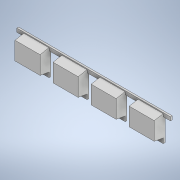
# Autodesk Inventor part: Buttons
Saved by Autodesk Inventor 2020 (Build 240168000, 168)
## iProperties
Created: 2022-03-19
Part Number: Buttons
Material: Типовые
Document SubType Name: Modeling
Designer: NoName
Density: 1 g/cm^3
Appearance: По умолчанию
Author: NoName
Autodesk Inventor part; units mm, degrees
ref_plane "YZ Plane" through (0, 0, 0) normal (1, 0, 0) x (0, 1, 0)
ref_plane "XZ Plane" through (0, 0, 0) normal (0, 1, 0) x (-1, 0, 0)
ref_plane "XY Plane" through (0, 0, 0) normal (0, 0, 1) x (1, 0, 0)
sketch "Эскиз1" plane through (0, 0, 0) normal (0, 0, 1) x (1, 0, 0)
  line L0 (0, 0) -> (5.6, 0)
  line L1 (5.6, 0) -> (5.6, 6)
  line L2 (5.6, 6) -> (0, 6)
  line L3 (0, 6) -> (0, 0)
  line L4 (8.5, 0) -> (14.1, 0)
  line L5 (14.1, 0) -> (14.1, 6)
  line L6 (14.1, 6) -> (8.5, 6)
  line L7 (8.5, 6) -> (8.5, 0)
  line L8 (17, 0) -> (22.6, 0)
  line L9 (22.6, 0) -> (22.6, 6)
  line L10 (22.6, 6) -> (17, 6)
  line L11 (17, 6) -> (17, 0)
  line L12 (25.5, 0) -> (31.1, 0)
  line L13 (31.1, 0) -> (31.1, 6)
  line L14 (31.1, 6) -> (25.5, 6)
  line L15 (25.5, 6) -> (25.5, 0)
  line L16 (5.6, 6) -> (8.5, 6)
  line L17 (14.1, 6) -> (17, 6)
  line L18 (22.6, 6) -> (25.5, 6)
  line L19 (22.6, 5.2) -> (25.5, 5.2)
  line L20 (17, 5.2) -> (14.1, 5.2)
  line L21 (8.5, 5.2) -> (5.6, 5.2)
  line L22 (0, 5.2) -> (-1.6, 5.2)
  line L23 (-1.6, 5.2) -> (-1.6, 6)
  line L24 (-1.6, 6) -> (0, 6)
  line L25 (0, 6) -> (0, 5.2)
  line L26 (31.1, 5.2) -> (32.7, 5.2)
  line L27 (32.7, 5.2) -> (32.7, 6)
  line L28 (32.7, 6) -> (31.1, 6)
  line L29 (31.1, 6) -> (31.1, 5.2)
  dimension "d0" = 5.6
  dimension "d1" = 6
  dimension "d4" = 8.5
  dimension "d9" = 0.8
  dimension "d10" = 1.6
  constraints: 60 end point, 11 point on line, 6 parallel, 5 horizontal, 5 perpendicular, 4 collinear, 4 horizontal alignment, 23 other
  measures "d0" distance between parallel lines of L3 L1
  measures "d1" distance between parallel lines of L0 L2
  measures "d4" distance of L0.start L4.start
  measures "d9" distance between parallel lines of L16 L21
  measures "d10" distance between parallel lines of L3 L23
extrude "Выдавливание1" add sketch "Эскиз1" along normal blind 0.4
sketch "Эскиз2" plane through (0, 0, 0.4) normal (0, 0, 1) x (1, 0, 0)
  line L0 (0, 5.2) -> (0, 0) projected
  line L1 (5.6, 0) -> (5.6, 5.2) projected
  line L2 (0, 1.1) -> (5.6, 1.1)
  line L3 (5.6, 1.1) -> (5.6, 5.8)
  line L4 (5.6, 5.8) -> (0, 5.8)
  line L5 (0, 5.8) -> (0, 1.1)
  line L6 (8.5, 5.2) -> (8.5, 0) projected
  line L7 (14.1, 0) -> (14.1, 5.2) projected
  line L8 (8.5, 1.1) -> (14.1, 1.1)
  line L9 (14.1, 1.1) -> (14.1, 5.8)
  line L10 (14.1, 5.8) -> (8.5, 5.8)
  line L11 (8.5, 5.8) -> (8.5, 1.1)
  line L12 (17, 5.2) -> (17, 0) projected
  line L13 (22.6, 0) -> (22.6, 5.2) projected
  line L14 (17, 1.1) -> (22.6, 1.1)
  line L15 (22.6, 1.1) -> (22.6, 5.8)
  line L16 (22.6, 5.8) -> (17, 5.8)
  line L17 (17, 5.8) -> (17, 1.1)
  line L18 (25.5, 5.2) -> (25.5, 0) projected
  line L19 (31.1, 0) -> (31.1, 5.2) projected
  line L20 (25.5, 1.1) -> (31.1, 1.1)
  line L21 (31.1, 1.1) -> (31.1, 5.8)
  line L22 (31.1, 5.8) -> (25.5, 5.8)
  line L23 (25.5, 5.8) -> (25.5, 1.1)
  line L24 (0, 0) -> (5.6, 0) projected
  point P0 (25.5, 5)
  point P1 (17, 5)
  point P2 (8.5, 5)
  point P3 (0, 5)
  dimension "d13" = 1.1
  dimension "d14" = 4.7
  constraints: 32 end point, 14 point on line, 8 parallel, 4 horizontal, 4 perpendicular
  measures "d13" distance between parallel lines of L24 L2
  measures "d14" distance between parallel lines of L2 L4
extrude "Выдавливание2" add sketch "Эскиз2" along normal blind 2 contours L5 L4 L3 L1 L2 L0 | L11 L10 L9 L7 L8 L6 | L17 L16 L15 L13 L14 L12 | L23 L22 L21 L19 L20 L18
sketch "Эскиз3" plane through (0, 0, 0) normal (-1, 0, 0) x (0, 0, 1)
  line L0 (0.4, 1.1) -> (2.4, 1.45)
  line L1 (0, 5.2) -> (0, 0) projected
  line L2 (0, 0) -> (0.4, 0) projected
  line L3 (0.4, 1.1) -> (0.4, 0) projected
  line L4 (0.4, 1.1) -> (2.4, 1.1) projected
  line L5 (2.4, 5.8) -> (2.4, 1.1) projected
  line L6 (0.4, 5.2) -> (0.4, 5.8) projected
  line L7 (0, 5.2) -> (0.4, 5.2) projected
  line L8 (0.4, 1.1) -> (2.4, 1.1)
  line L9 (0.4, 5.8) -> (2.4, 5.8)
  line L10 (0.4, 5.8) -> (2.4, 5.45)
  line L11 (2.4, 1.1) -> (2.4, 5.8) projected
  line L12 (2.4, 1.45) -> (2.4, 1.1)
  line L13 (0.4, 5.8) -> (2.4, 5.8) projected
  line L14 (0.4, 6) -> (0.4, 5.2) projected
  line L15 (2.4, 5.8) -> (2.4, 1.1) projected
  line L16 (2.4, 5.45) -> (2.4, 5.8)
  point P0 (2, 5.8)
  point P1 (2, 5.6739)
  point P2 (2, 5.8)
  dimension "d18" = 4
  constraints: 12 end point, 2 point on line, 2 vertical, 1 collinear, 1 equal length, 1 horizontal, 1 other
  measures "d18" distance of L0.end L10.end
extrude "Выдавливание3" cut sketch "Эскиз3" against normal through all contours L0 L5 L4 | L10 L9 L5
